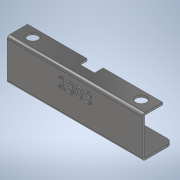
# Autodesk Inventor part: 0 零件
Saved by Autodesk Inventor 2020 (Build 240168000, 168)
## iProperties
Created: 2020-11-03
Part Number: 0 零件
Material: 不鏽鋼
Document SubType Name: Sheet Metal
Designer: p2013
Density: 8 g/cm^3
Appearance: 不鏽鋼 - 疏刷
Sheet Metal Rule: 預設 mm (_M)
Sheet Metal Width: 79.065 mm
Sheet Metal Length: 124.700 mm
Sheet Metal Area: 9859.356 mm^2
Flat Pattern Width: 7.90646 cm
Flat Pattern Length: 12.47 cm
Flat Pattern Area: 98.5936 cm^2
Author: p2013
Autodesk Inventor part; units mm, degrees
ref_plane "YZ Plane" through (0, 0, 0) normal (1, 0, 0) x (0, 1, 0)
ref_plane "XZ Plane" through (0, 0, 0) normal (0, 1, 0) x (-1, 0, 0)
ref_plane "XY Plane" through (0, 0, 0) normal (0, 0, 1) x (1, 0, 0)
sketch "草圖1" plane through (0, 0, 0) normal (0, 0, 1) x (1, 0, 0)
  line L0 (0, -42.8) -> (-53.4141, -42.8) construction
  line L1 (0, -42.8) -> (0, 26.5671) construction
  line L2 (-62.35, 33.5) -> (-7.5, 33.5)
  line L3 (62.35, 33.5) -> (62.35, -42.8)
  line L4 (62.35, -42.8) -> (-62.35, -42.8)
  line L5 (-62.35, -42.8) -> (-62.35, 33.5)
  line L6 (-62.35, 16.5) -> (62.35, 16.5)
  line L7 (-62.35, -16.5) -> (62.35, -16.5)
  line L8 (-62.35, 16.5) -> (62.35, -16.5) construction
  circle A0 centre (-50, 26) radius 5
  line L9 (0, 4) -> (0, 4) construction
  circle A1 centre (50, 26) radius 5
  line L10 (-16.3, 12) -> (17.6086, 12) construction
  line L11 (17.6086, 12) -> (17.6086, 1.2491) construction
  line L12 (17.6086, 1.2491) -> (-16.3, 1.2491) construction
  line L13 (-16.3, 1.2491) -> (-16.3, 12) construction
  line L14 (7.5, 33.5) -> (0, 33.5) construction
  line L15 (-7.5, 33.5) -> (-7.5, 25.5)
  line L16 (-7.5, 25.5) -> (7.5, 25.5)
  line L17 (7.5, 25.5) -> (7.5, 33.5)
  line L18 (0, 33.5) -> (-7.5, 33.5) construction
  line L19 (7.5, 33.5) -> (62.35, 33.5)
  line L20 (-7.5, 33.5) -> (7.5, 33.5) construction
  arc A2 (-60.8627, 16.1064) -> (-60.85, 16.5) centre (-66.9333, 16.5) ccw
  line L21 (-62.35, 12.5) -> (-61.2545, 14.7472)
  line L22 (-61.2545, 18.2528) -> (-62.35, 20.5)
  arc A3 (-61.2545, 14.7472) -> (-61.2545, 18.2528) centre (-64.85, 16.5) ccw
  line L23 (62.35, 12.5) -> (61.2545, 14.7472)
  line L24 (61.2545, 18.2528) -> (62.35, 20.5)
  arc A4 (61.2545, 18.2528) -> (61.2545, 14.7472) centre (64.85, 16.5) ccw
  line L25 (-15.2508, 1.8313) -> (-15.2508, 3.7608)
  line L26 (-15.2508, 3.7608) -> (-13.1305, 3.7608)
  line L27 (-13.1305, 3.7608) -> (-13.1305, 9.4395)
  line L28 (-13.1305, 9.4395) -> (-14.972, 9.4395)
  line L29 (-14.972, 9.4395) -> (-14.972, 10.9142)
  spline S0 degree 2 poles (-14.972, 10.9142) (-13.512, 11.1856) (-12.4996, 11.8313) knots 0 0 0 1 1 1
  line L30 (-12.4996, 11.8313) -> (-11.6191, 11.8313)
  line L31 (-11.6191, 11.8313) -> (-10.7461, 10.9582)
  line L32 (-10.7461, 10.9582) -> (-10.7461, 3.7608)
  line L33 (-10.7461, 3.7608) -> (-8.9486, 3.7608)
  line L34 (-8.9486, 3.7608) -> (-8.9486, 1.8313)
  line L35 (-8.9486, 1.8313) -> (-15.2508, 1.8313)
  spline S1 degree 2 poles (-4.3851, 1.6405) (-6.6081, 1.6405) (-7.804, 3.0418) knots 0 0 0 1 1 1
  line L36 (-7.804, 3.0418) -> (-6.7035, 4.5385)
  spline S2 degree 2 poles (-6.7035, 4.5385) (-5.669, 3.5774) (-4.6272, 3.5774) knots 0 0 0 1 1 1
  spline S3 degree 2 poles (-4.6272, 3.5774) (-3.9156, 3.5774) (-3.512, 3.8709) knots 0 0 0 1 1 1
  spline S4 degree 2 poles (-3.512, 3.8709) (-3.0938, 4.1643) (-3.0938, 4.7806) knots 0 0 0 1 1 1
  spline S5 degree 2 poles (-3.0938, 4.7806) (-3.0938, 5.4116) (-4.165, 6.0866) (-4.5539, 6.0205) knots 0 0 0 1 2 2 2
  line L37 (-4.5539, 6.0205) -> (-5.647, 6.9596)
  line L38 (-5.647, 6.9596) -> (-5.647, 7.774)
  spline S6 degree 2 poles (-5.647, 7.774) (-4.4218, 7.774) (-3.402, 8.449) (-3.402, 9.08) knots 0 0 0 1 2 2 2
  spline S7 degree 2 poles (-3.402, 9.08) (-3.402, 10.1365) (-4.5465, 10.1365) knots 0 0 0 1 1 1
  spline S8 degree 2 poles (-4.5465, 10.1365) (-5.3902, 10.1365) (-6.3293, 9.3074) knots 0 0 0 1 1 1
  line L39 (-6.3293, 9.3074) -> (-7.5399, 10.7674)
  spline S9 degree 2 poles (-7.5399, 10.7674) (-6.0726, 12) (-2.8517, 12) (-1.942, 11.281) knots 0 0 0 1 2 2 2
  spline S10 degree 2 poles (-1.942, 11.281) (-1.0175, 10.5693) (-1.0175, 9.2487) knots 0 0 0 1 1 1
  spline S11 degree 2 poles (-1.0175, 9.2487) (-1.0175, 7.6933) (-2.6096, 6.9817) knots 0 0 0 1 1 1
  spline S12 degree 2 poles (-2.6096, 6.9817) (-1.7365, 6.7175) (-0.6947, 5.4776) (-0.6947, 4.5532) knots 0 0 0 1 2 2 2
  spline S13 degree 2 poles (-0.6947, 4.5532) (-0.6947, 3.2106) (-1.7659, 2.4182) knots 0 0 0 1 1 1
  spline S14 degree 2 poles (-1.7659, 2.4182) (-2.8297, 1.6405) (-4.3851, 1.6405) knots 0 0 0 1 1 1
  spline S15 degree 2 poles (6.7154, 2.9978) (5.7616, 1.6405) (2.5188, 1.6405) (0.5966, 4.3551) (0.5966, 9.3881) (2.5188, 12) (5.7616, 12) (7.6692, 9.3734) (7.6692, 4.3551) (6.7154, 2.9978) knots 0 0 0 1 2 3 4 5 6 7 8 8 8
  spline S16 degree 2 poles (3.1938, 4.2304) (3.5386, 3.4967) (4.7418, 3.4967) (5.4168, 4.9714) (5.4168, 8.1775) (5.05, 9.6963) (4.5291, 10.1805) (3.7514, 10.1805) (3.2158, 9.6963) (2.8489, 8.1775) (2.8489, 4.9714) (3.1938, 4.2304) knots 0 0 0 1 2 3 4 5 6 7 8 9 10 10 10
  spline S17 degree 2 poles (11.9612, 1.6405) (9.7382, 1.6405) (8.5423, 3.0418) knots 0 0 0 1 1 1
  line L40 (8.5423, 3.0418) -> (9.6428, 4.5385)
  spline S18 degree 2 poles (9.6428, 4.5385) (10.6773, 3.5774) (11.7191, 3.5774) knots 0 0 0 1 1 1
  spline S19 degree 2 poles (11.7191, 3.5774) (12.4307, 3.5774) (12.8343, 3.8709) knots 0 0 0 1 1 1
  spline S20 degree 2 poles (12.8343, 3.8709) (13.2525, 4.1643) (13.2525, 4.7806) knots 0 0 0 1 1 1
  spline S21 degree 2 poles (13.2525, 4.7806) (13.2525, 5.4116) (12.1813, 6.0866) (11.7924, 6.0205) knots 0 0 0 1 2 2 2
  line L41 (11.7924, 6.0205) -> (10.6993, 6.9596)
  line L42 (10.6993, 6.9596) -> (10.6993, 7.774)
  spline S22 degree 2 poles (10.6993, 7.774) (11.9245, 7.774) (12.9443, 8.449) (12.9443, 9.08) knots 0 0 0 1 2 2 2
  spline S23 degree 2 poles (12.9443, 9.08) (12.9443, 10.1365) (11.7998, 10.1365) knots 0 0 0 1 1 1
  spline S24 degree 2 poles (11.7998, 10.1365) (10.9561, 10.1365) (10.0169, 9.3074) knots 0 0 0 1 1 1
  line L43 (10.0169, 9.3074) -> (8.8064, 10.7674)
  spline S25 degree 2 poles (8.8064, 10.7674) (10.2737, 12) (13.4946, 12) (14.4043, 11.281) knots 0 0 0 1 2 2 2
  spline S26 degree 2 poles (14.4043, 11.281) (15.3288, 10.5693) (15.3288, 9.2487) knots 0 0 0 1 1 1
  spline S27 degree 2 poles (15.3288, 9.2487) (15.3288, 7.6933) (13.7367, 6.9817) knots 0 0 0 1 1 1
  spline S28 degree 2 poles (13.7367, 6.9817) (14.6098, 6.7175) (15.6516, 5.4776) (15.6516, 4.5532) knots 0 0 0 1 2 2 2
  spline S29 degree 2 poles (15.6516, 4.5532) (15.6516, 3.2106) (14.5804, 2.4182) knots 0 0 0 1 1 1
  spline S30 degree 2 poles (14.5804, 2.4182) (13.5166, 1.6405) (11.9612, 1.6405) knots 0 0 0 1 1 1
  point P0 (0, 0)
  point P1 (0, 0)
  point P2 (40.65, 33.5)
  point P3 (29.0517, 33.5)
  point P4 (-60.4, 16.5)
  dimension "d0" = 124.7
  dimension "d1" = 26.3
  dimension "d2" = 33
  dimension "d3" = 17
  dimension "d11" = 10
  dimension "d15" = 0
  dimension "d18" = 100
  dimension "d36" = 4.5
  dimension "d53" = 7.5
  dimension "d54" = 15
  dimension "d55" = 8
  dimension "d56" = 8
  dimension "d57" = 1.5
  dimension "d58" = 16.3
  dimension "d59" = 4
  constraints: 42 end point, 16 point on line, 7 horizontal, 7 parallel, 7 perpendicular, 7 point on circle, 7 symmetric about line, 5 centre point, 2 midpoint, 2 tangent, 2 vertical, 1 coincident, 1 horizontal alignment, 6 other
  measures "d0" distance between parallel lines of L3 L5
  measures "d1" distance between parallel lines of L7 L4
  measures "d2" distance between parallel lines of L6 L7
  measures "d3" distance between parallel lines of L6 L2
  measures "d11" diameter of A0
  measures "d15" distance of L9.end L9.start
  measures "d18" distance of A1.centre A0.centre
  measures "d36" distance between parallel lines of L6 L10
  measures "d53" distance from line of A1.centre L2
  measures "d54" distance between parallel lines of L17 L15
  measures "d55" distance between parallel lines of L14 L16
  measures "d56" distance of L22.end L21.start
  measures "d57" distance edge to line of A2 L5
  measures "d58" distance from line of L1 L10.start
  measures "d59" radius of A3
extrude "擠出1" add sketch "草圖1" along normal blind 2 contours L2 L15 L16 L17 L19 L3 L24 A4 L6 A3 L22 L5 | L22 A3 L6 L5 | L6 A3 L21 L5 | L21 A3 L6 A4 L23 L3 L7 L5 | L7 L3 L4 L5 | A4 L24 L3 L6 | L6 L3 L23 A4 | L25 L26 L27 L28 L29 S0 L30 L31 L32 L33 L34 L35 | S1 L36 S2 S3 S4 S5 L37 L38 S6 S7 S8 L39 S9 S10 S11 S12 S13 S14 | S15 | S16 | S17 L40 S18 S19 S20 S21 L41 L42 S22 S23 S24 L43 S25 S26 S27 S28 S29 S30
extrude "擠出3" cut sketch "草圖1" along normal up to surface (2 mm away) contours L25 L26 L27 L28 L29 S0 L30 L31 L32 L33 L34 L35 | S1 L36 S2 S3 S4 S5 L37 L38 S6 S7 S8 L39 S9 S10 S11 S12 S13 S14 | S15 | S17 L40 S18 S19 S20 S21 L41 L42 S22 S23 S24 L43 S25 S26 S27 S28 S29 S30
sketch "草圖4" plane through (0, 0, 2) normal (0, 0, 1) x (1, 0, 0)
  spline S0 degree 2 poles (6.7154, 2.9978) (5.7616, 1.6405) (2.5188, 1.6405) (0.5966, 4.3551) (0.5966, 9.3881) (2.5188, 12) (5.7616, 12) (7.6692, 9.3734) (7.6692, 4.3551) (6.7154, 2.9978) knots 0 0 0 0.125 0.25 0.375 0.5 0.625 0.75 0.875 1 1 1 projected
  spline S1 degree 2 poles (3.1938, 4.2304) (3.5386, 3.4967) (4.7418, 3.4967) (5.4168, 4.9714) (5.4168, 8.1775) (5.05, 9.6963) (4.5291, 10.1805) (3.7514, 10.1805) (3.2158, 9.6963) (2.8489, 8.1775) (2.8489, 4.9714) (3.1938, 4.2304) knots 0 0 0 0.1 0.2 0.3 0.4 0.5 0.6 0.7 0.8 0.9 1 1 1 projected
  line L0 (0, 10.0218) -> (7.4981, 2.5237)
  line L1 (0.7071, 10.7289) -> (8.2052, 3.2308)
  line L2 (0, 10.0218) -> (0.7071, 10.7289)
  line L3 (7.4981, 2.5237) -> (8.2052, 3.2308)
  line L4 (0, 48.76) -> (0, -58.06) projected
  point P0 (0, 0)
  point P1 (7.287, 4.149)
  point P2 (5.4061, 6.0299)
  point P3 (5.2545, 4.7673)
  point P4 (6.8382, 3.1836)
  point P5 (2.9496, 8.4864)
  point P6 (1.2457, 10.1903)
  point P7 (0.8573, 9.1645)
  point P8 (2.8559, 7.1659)
  dimension "d45" = 45
  dimension "d46" = 1
  dimension "d47" = 7.4981
  dimension "d48" = 10.0218
  constraints: 8 end point, 2 parallel, 1 perpendicular, 1 point on line, 1 vertical alignment, 2 other
  measures "d45" angle of L4 L1
  measures "d46" distance between parallel lines of L0 L1
  measures "d47" horizontal distance of L1.start L1.end
  measures "d48" distance of point (0, 0) L0.start
extrude "擠出4" add sketch "草圖4" against normal up to surface (2 mm away) contours S0 L1 S1 L0 | L0 S1 L1 S0
bend part "折彎零件1" radius 0.5 angle 90 line through (-62.35, 16.5, 0) along (1, 0, 0) centre toward (0, 0, -1) moving side (0, 1, 0) both sides no
bend part "折彎零件2" radius 0.5 angle 90 line through (-62.35, -16.5, 0) along (1, 0, 0) centre toward (0, 0, -1) moving side (0, -1, 0) both sides no
fillet "圓角1" radius 5 2 edges at (62.35, -18, -26.0146) (-62.35, -18, -26.0146)
